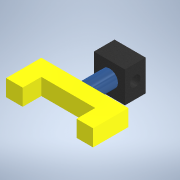
# Autodesk Inventor part: HOLDER
Saved by Autodesk Inventor 2021 (Build 250183000, 183)
## iProperties
Created: 2021-07-24
Part Number: HOLDER
Material: Generic
Document SubType Name: Modeling
Designer: aksha
Density: 1 g/cm^3
Appearance: Default
Author: aksha
Autodesk Inventor part; units mm, degrees
ref_plane "YZ Plane" through (0, 0, 0) normal (1, 0, 0) x (0, 1, 0)
ref_plane "XZ Plane" through (0, 0, 0) normal (0, 1, 0) x (-1, 0, 0)
ref_plane "XY Plane" through (0, 0, 0) normal (0, 0, 1) x (1, 0, 0)
sketch "Sketch1" plane through (0, 0, 0) normal (0, 0, 1) x (1, 0, 0)
  line L0 (-80.9183, 81.3988) -> (69.0817, 81.3988)
  line L1 (69.0817, 81.3988) -> (69.0817, -68.6012)
  line L2 (69.0817, -68.6012) -> (-80.9183, -68.6012)
  line L3 (-80.9183, -68.6012) -> (-80.9183, 81.3988)
  line L4 (-80.9183, 81.3988) -> (69.0817, -68.6012) construction
  line L5 (69.0817, 81.3988) -> (-80.9183, -68.6012) construction
  point P0 (0, 0)
  point P1 (-5.9183, 6.3988)
  dimension "d0" = 150
  dimension "d1" = 150
  constraints: 12 end point, 2 midpoint, 2 parallel, 1 horizontal, 1 perpendicular
  measures "d0" distance of L1.end L2.end
  measures "d1" distance of L0.end L1.end
extrude "Extrusion1" add sketch "Sketch1" along normal blind 100
sketch "Sketch2" plane through (0, 0, 100) normal (0, 0, 1) x (1, 0, 0)
  circle A0 centre (-4.4387, 8.6963) radius 40
  point P0 (0, 0)
  dimension "d4" = 80
  constraints: 1 centre point
  measures "d4" diameter of A0
extrude "Extrusion2" add sketch "Sketch2" along normal blind 120
sketch "Sketch3" plane through (-4.4387, 8.6963, 220) normal (0, 0, 1) x (1, 0, 0)
  line L0 (-210, 40) -> (210, 40)
  line L1 (210, 40) -> (210, -40)
  line L2 (210, -40) -> (-210, -40)
  line L3 (-210, -40) -> (-210, 40)
  circle A0 centre (0, 0) radius 40 projected
  line L4 (-210, 40) -> (210, -40) construction
  line L5 (210, 40) -> (-210, -40) construction
  point P0 (4.4387, -8.6963)
  dimension "d7" = 420
  dimension "d8" = 80
  constraints: 12 end point, 2 midpoint, 2 parallel, 1 horizontal, 1 perpendicular
  measures "d7" distance of L1.end L2.end
  measures "d8" distance of L0.end L1.end
extrude "Extrusion3" add sketch "Sketch3" along normal blind 80
sketch "Sketch4" plane through (-4.4387, 8.6963, 300) normal (0, 0, 1) x (1, 0, 0)
  line L0 (210, 40) -> (-210, 40) projected
  line L1 (-210, -40) -> (210, -40) projected
  line L2 (-210, 40) -> (-130, 40)
  line L3 (-130, 40) -> (-130, -40)
  line L4 (-130, -40) -> (-210, -40)
  line L5 (-210, -40) -> (-210, 40)
  line L6 (210, -40) -> (210, 40) projected
  line L7 (210, 40) -> (130, 40)
  line L8 (130, 40) -> (130, -40)
  line L9 (130, -40) -> (210, -40)
  line L10 (210, -40) -> (210, 40)
  point P0 (4.4387, -8.6963)
  point P1 (130, 40)
  dimension "d11" = 80
  dimension "d12" = 80
  constraints: 16 end point, 4 parallel, 2 horizontal, 2 perpendicular, 2 point on line
  measures "d11" distance of L3.end L4.end
  measures "d12" distance of L9.end L8.end
extrude "Extrusion4" add sketch "Sketch4" along normal blind 90 contours L6 L1 L8 L0 | L3 L1 L5 L0
sketch "Sketch5" plane through (69.0817, -68.6012, 0) normal (1, 0, 0) x (0, 0, -1)
  circle A0 centre (-49.808, 76.4656) radius 25
  point P0 (0, 68.6012)
  dimension "d15" = 50
  constraints: 1 centre point
  measures "d15" diameter of A0
extrude "Extrusion5" cut sketch "Sketch5" against normal blind 500
body "Solid1"
